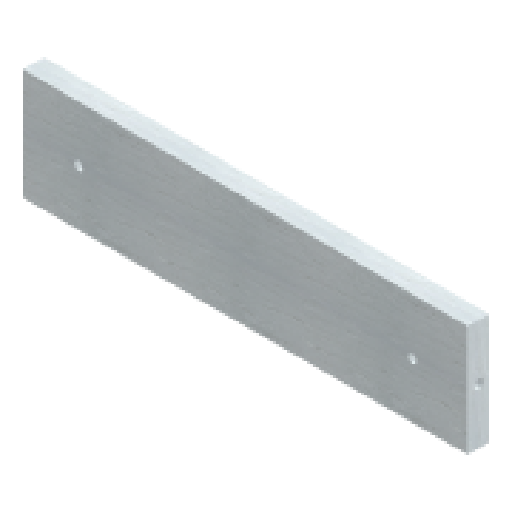
# Autodesk Inventor part: A
Saved by Autodesk Inventor 2024 (Build 280153000, 153)
## iProperties
Created: 2024-03-20
Part Number: A
Material: Generic
Document SubType Name: Modeling
Designer: marco
Density: 1 g/cm^3
Appearance: Wood - Painted White
Author: marco
Autodesk Inventor part; units mm, degrees
ref_plane "YZ Plane" through (0, 0, 0) normal (1, 0, 0) x (0, 1, 0)
ref_plane "XZ Plane" through (0, 0, 0) normal (0, 1, 0) x (-1, 0, 0)
ref_plane "XY Plane" through (0, 0, 0) normal (0, 0, 1) x (1, 0, 0)
sketch "Sketch1" plane through (0, 0, 0) normal (0, 0, 1) x (1, 0, 0)
  line L0 (-200, -50) -> (200, -50)
  line L1 (200, -50) -> (200, 50)
  line L2 (200, 50) -> (-200, 50)
  line L3 (-200, 50) -> (-200, -50)
  line L4 (-200, -50) -> (200, 50) construction
  line L5 (200, -50) -> (-200, 50) construction
  point P0 (0, 0)
  dimension "d0" = 400
  dimension "d1" = 100
  constraints: 12 end point, 2 midpoint, 2 parallel, 1 horizontal, 1 perpendicular
  measures "d0" distance of L2.end L1.end
  measures "d1" distance of L1.end L0.end
extrude "Extrusion1" add sketch "Sketch1" along normal blind 9.5 and the other way blind 9.5
sketch "Sketch2" plane through (0, 0, 9.5) normal (0, 0, 1) x (1, 0, 0)
  line L0 (-200, 50) -> (-200, -50) projected
  line L1 (-200, 0) -> (-150, 0)
  line L2 (200, -50) -> (200, 50) projected
  line L3 (200, 0) -> (150, 0)
  circle A0 centre (-150, 0) radius 4
  circle A1 centre (150, 0) radius 4
  point P0 (0, 0)
  dimension "d6" = 50
  dimension "d7" = 50
  dimension "d8" = 8
  dimension "d9" = 8
  constraints: 4 end point, 2 centre point, 2 coincident, 2 horizontal, 2 midpoint
  measures "d6" distance of L1.start L1.end
  measures "d7" distance of L3.start L3.end
  measures "d8" diameter of A0
  measures "d9" diameter of A1
extrude "Extrusion2" cut sketch "Sketch2" against normal blind 11
sketch "Sketch3" plane through (200, -50, 9.5) normal (1, 0, 0) x (0, 0, -1)
  circle A0 centre (9.5, 50) radius 4
  dimension "d12" = 8
  constraints: 1 centre point, 1 coincident
  measures "d12" diameter of A0
extrude "Extrusion3" cut sketch "Sketch3" against normal blind 11
sketch "Sketch4" plane through (-200, -50, 9.5) normal (-1, 0, 0) x (0, 0, 1)
  circle A0 centre (-9.5, 50) radius 4
  dimension "d15" = 8
  constraints: 1 centre point, 1 coincident
  measures "d15" diameter of A0
extrude "Extrusion4" cut sketch "Sketch4" against normal blind 11
body "Solid1"
